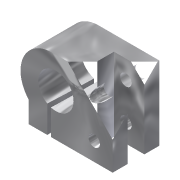
# Autodesk Inventor part: suporte-eixo
Saved by Autodesk Inventor 2015 (Build 190159000, 159)
## iProperties
Created: 2016-08-10
Part Number: suporte-eixo
Material: Ogólny
Document SubType Name: Modeling
Designer: EriveltonDell
Density: 1 g/cm^3
Appearance: Aluminum - Polished
Mass: 33.9428 g
Surface Area: 112.837 cm^2
Volume: 33.9428 cm^3
Author: EriveltonDell
Autodesk Inventor part; units mm, degrees
ref_plane "YZ Plane" through (0, 0, 0) normal (1, 0, 0) x (0, 1, 0)
ref_plane "XZ Plane" through (0, 0, 0) normal (0, 1, 0) x (-1, 0, 0)
ref_plane "XY Plane" through (0, 0, 0) normal (0, 0, 1) x (1, 0, 0)
sketch "Sketch1" plane through (0, 0, 0) normal (0, 1, 0) x (-1, 0, 0)
  line L0 (50, 0) -> (50, 40)
  line L1 (50, 40) -> (0, 40)
  line L2 (0, 40) -> (0, 0)
  line L3 (0, 0) -> (10, 0)
  line L4 (10, 0) -> (10, 10)
  line L5 (10, 10) -> (10, 30)
  circle A0 centre (10, 30) radius 3.1
  circle A1 centre (10, 10) radius 3.1
  line L6 (45.5, 0) -> (45.5, 11.4783)
  line L7 (0, 0) -> (33.5, 0)
  line L8 (35.5, 0) -> (35.5, 18.6699)
  line L9 (50, 40) -> (45.5, 40)
  line L10 (45.5, 40) -> (45.5, 35.5)
  line L11 (45.5, 35.5) -> (45.5, 34.5217)
  line L12 (45.5, 23) -> (33, 23)
  arc A2 (45.5, 11.4783) -> (33, 40) centre (33, 23) ccw
  line L13 (0, 0) -> (33.5, 0)
  line L14 (35.5, 0) -> (45.5, 0)
  line L15 (33.5, 0) -> (33.5, 18.0251)
  line L16 (0, 0) -> (33.5, 0)
  line L17 (35.5, 0) -> (45.5, 0)
  line L18 (33, 23) -> (28, 23)
  line L19 (33, 23) -> (38, 23)
  arc A3 (35.5, 18.6699) -> (38, 23) centre (33, 23) ccw
  arc A4 (28, 23) -> (33.5, 18.0251) centre (33, 23) ccw
  dimension "d0" = 50
  dimension "d1" = 40
  dimension "d2" = 10
  dimension "d3" = 10
  dimension "d4" = 20
  dimension "d5" = 6.2
  dimension "d6" = 6.2
  dimension "d7" = 45.5
  dimension "d8" = 35.5
  dimension "d9" = 4.5
  dimension "d10" = 4.5
  dimension "d13" = 12.5
  dimension "d14" = 12.5
  dimension "d15" = 2
  constraints: 40 end point, 9 perpendicular, 7 point on circle, 5 centre point, 4 horizontal, 4 point on line, 3 coincident, 3 parallel, 1 tangent, 1 vertical
  measures "d0" distance of L1.end L0.end
  measures "d1" distance of L0.end L0.start
  measures "d2" distance of L2.end L3.end
  measures "d3" distance of L3.end L4.end
  measures "d4" distance of L4.end L5.end
  measures "d5" diameter of A0
  measures "d6" diameter of A1
  measures "d7" distance of L6.start L2.end
  measures "d8" distance of L2.end L8.start
  measures "d9" distance of L0.end L9.end
  measures "d10" distance of L9.end L10.end
  measures "d13" distance of L12.start L10.end
  measures "d14" distance of L12.start L12.end
  measures "d15" distance of L7.end L8.start
extrude "Extrusion1" add sketch "Sketch1" along normal blind 25.4 contours A2 L6 L14 L8 A3 L12 L18 A4 L15 L7 L3 L2 L1
sketch "Sketch2" plane through (-33, 0, 40) normal (0, 0, 1) x (1, 0, 0)
  line L0 (33, 0) -> (33, 8.2)
  line L1 (33, 0) -> (33, 25.4) projected
  line L2 (33, 8.2) -> (16.5, 8.2)
  line L3 (16.5, 8.2) -> (16.5, 17.2)
  line L4 (16.5, 17.2) -> (33, 17.2)
  line L5 (33, 17.2) -> (33, 8.2)
  dimension "d18" = 8.2
  dimension "d19" = 16.5
  dimension "d20" = 9
  constraints: 10 end point, 2 perpendicular, 2 point on line, 1 collinear, 1 vertical
  measures "d18" distance of L0.start L0.end
  measures "d19" distance of L0.end L2.end
  measures "d20" distance of L2.end L3.end
extrude "Extrusion2" cut sketch "Sketch2" against normal through all
sketch "Sketch6" plane through (-28, 0, 23) normal (0, 0, -1) x (-1, 0, 0)
  line L0 (10, 25.4) -> (5.5, 25.4)
  line L1 (0, 25.4) -> (5.5, 25.4) projected
  line L2 (5.5, 25.4) -> (7.7222, 0)
  line L3 (7.5, 0) -> (17.5, 0) projected
  line L4 (5.5, 25.4) -> (30.997, 25.4) construction
  line L5 (7.5, 0) -> (8.3716, -9.9619)
  line L6 (7.5, 0) -> (17.5, 0) construction
  line L7 (15.2207, 20.7519) -> (-3.707, 19.0959)
  line L8 (-3.707, 19.0959) -> (-1.0923, -10.7899)
  line L9 (-1.0923, -10.7899) -> (8.3716, -9.9619)
  line L10 (8.3716, -9.9619) -> (5.7569, 19.9239)
  line L11 (8.3716, -9.9619) -> (38.3716, -9.9619) construction
  line L12 (8.3716, -9.9619) -> (5.7569, 19.9239)
  line L13 (-1.0923, -10.7899) -> (-3.707, 19.0959)
  line L14 (-1.0923, -10.7899) -> (28.9077, -10.7899) construction
  line L15 (-3.707, 19.0959) -> (5.7569, 19.9239)
  line L16 (5.7569, 19.9239) -> (8.3716, -9.9619)
  point P0 (-28, 0)
  dimension "d35" = 85
  dimension "d36" = 10
  dimension "d37" = 85
  dimension "d43" = 30
  dimension "d44" = 90
  dimension "d45" = 30
  dimension "d47" = 30
  dimension "d48" = 95
  dimension "d49" = 9.5
  constraints: 30 end point, 4 equal length, 4 horizontal, 3 collinear, 2 perpendicular, 1 point on line
  measures "d35" angle of L2 L4
  measures "d36" distance of L3.start L5.end
  measures "d37" angle of L5 L6
  measures "d43" distance of L7.end L8.end
  measures "d44" angle of L8 L7
  measures "d45" distance of L5.end L10.end
  measures "d47" distance of L8.end L7.end
  measures "d48" angle of L14 L13
  measures "d49" distance of L7.end L10.end
revolve "Revolution2" cut sketch "Sketch6" angle 360 about axis through (-36.3716, -9.9619, 23) along (0.0871557, 0.9961947, 0) contours L10 L5 L9 L8 L7
body "Solid1"
